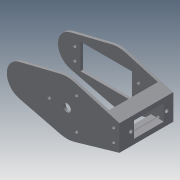
# Autodesk Inventor part: zakonceni_ramene
Saved by Autodesk Inventor 2013 (Build 170138000, 138)
## iProperties
Created: 2013-05-11
Part Number: zakonceni_ramene
Material: Generic
Document SubType Name: Modeling
Designer: idle-rug
Density: 1 g/cm^3
Author: idle-rug
Autodesk Inventor part; units mm, degrees
ref_plane "YZ Plane" through (0, 0, 0) normal (1, 0, 0) x (0, 1, 0)
ref_plane "XZ Plane" through (0, 0, 0) normal (0, 1, 0) x (-1, 0, 0)
ref_plane "XY Plane" through (0, 0, 0) normal (0, 0, 1) x (1, 0, 0)
sketch "Sketch1" plane through (0, 0, 0) normal (0, 1, 0) x (-1, 0, 0)
  circle A0 centre (0, 0) radius 21
  line L0 (-21, 0) -> (-41, 0)
  line L1 (-41, 0) -> (-41, -10)
  line L2 (-41, -10) -> (-18.466185, -10)
  line L3 (-41, 0) -> (-41, 10)
  line L4 (-41, 10) -> (-18.466185, 10)
  line L5 (-41, 10) -> (-5.8359, 20.17281)
  line L6 (-41, -10) -> (-5.8359, -20.17281)
  arc A1 (-5.8359, 20.17281) -> (-5.8359, -20.17281) centre (0, 0) ccw
  dimension "d0" = 42
  dimension "d1" = 20
  dimension "d2" = 10
  dimension "d3" = 10
  constraints: 14 end point, 7 point on circle, 4 tangent, 3 perpendicular, 2 centre point, 1 coincident, 1 horizontal, 1 parallel
  measures "d0" diameter of A0
  measures "d1" distance of L0.start L0.end
  measures "d2" distance of L0.end L1.end
  measures "d3" distance of L0.end L3.end
extrude "Extrusion1" add sketch "Sketch1" along normal blind 2
sketch "Sketch2" plane through (0, 0, 0) normal (0, -1, 0) x (1, 0, 0)
  arc A0 (5.8359, 20.17281) -> (5.8359, -20.17281) centre (0, 0) ccw
  circle A1 centre (0, 0) radius 3
  dimension "d11" = 6
  constraints: 1 centre point, 1 coincident
  measures "d11" diameter of A1
extrude "Extrusion2" cut sketch "Sketch2" against normal blind 2
sketch "Sketch3" plane through (0, 2, 0) normal (0, 1, 0) x (1, 0, 0)
  line L0 (5.8359, -20.17281) -> (41, -10)
  line L1 (41, -10) -> (41, 10)
  line L2 (41, 10) -> (5.8359, 20.17281)
  line L3 (39, 0) -> (39, 10.578591)
  line L4 (39, 0) -> (39, -10.578591)
  line L5 (41, 10) -> (41, -10)
  line L6 (39, -10.578591) -> (41, -10)
  line L7 (39, 10.578591) -> (41, 10)
  constraints: 10 end point, 3 collinear, 2 point on line, 1 parallel
extrude "Extrusion3" add sketch "Sketch3" along normal blind 48
sketch "Sketch4" plane through (0, 50, 0) normal (0, 1, 0) x (1, 0, 0)
  line L0 (41, -10) -> (41, 10)
  line L1 (39, -10.578591) -> (41, -10)
  circle A0 centre (0, 0) radius 21
  line L2 (41, 10) -> (5.8359, 20.17281)
  line L3 (41, -10) -> (5.8359, -20.17281)
  line L4 (41, 10) -> (41, -10)
  circle A1 centre (0, 0) radius 3
  dimension "d17" = 42
  dimension "d18" = 6
  constraints: 6 end point, 2 centre point, 2 coincident, 2 collinear, 2 point on circle, 1 tangent
  measures "d17" diameter of A0
  measures "d18" diameter of A1
extrude "Extrusion4" add sketch "Sketch4" along normal blind 2
sketch "Sketch5" plane through (41, 0, 10) normal (1, 0, 0) x (0, 0, -1)
  line L0 (10, 26) -> (10, 42)
  line L1 (10, 42) -> (10, 10)
  line L2 (10, 42) -> (10, 39.95)
  line L3 (10, 10) -> (10, 12.05)
  circle A0 centre (10, 39.95) radius 1.5
  circle A1 centre (10, 12.05) radius 1.5
  line L4 (10, 12.05) -> (10, 14.4)
  line L5 (10, 39.95) -> (10, 37.6)
  line L6 (10, 37.6) -> (10, 14.4)
  line L7 (16.2, 14.4) -> (3.8, 14.4)
  line L8 (3.8, 14.4) -> (3.8, 37.6)
  line L9 (3.8, 37.6) -> (16.2, 37.6)
  line L10 (16.2, 37.6) -> (16.2, 14.4)
  line L11 (16.2, 14.4) -> (3.8, 37.6) construction
  line L12 (3.8, 14.4) -> (16.2, 37.6) construction
  point P0 (10, 0)
  dimension "d23" = 2.05
  dimension "d24" = 2.05
  dimension "d25" = 3
  dimension "d26" = 3
  dimension "d27" = 2.35
  dimension "d28" = 2.35
  dimension "d29" = 12.4
  constraints: 26 end point, 4 point on line, 2 centre point, 2 coincident, 2 collinear, 2 midpoint, 2 parallel, 1 horizontal, 1 perpendicular
  measures "d23" distance of L0.end L2.end
  measures "d24" distance of L1.end L3.end
  measures "d25" diameter of A0
  measures "d26" diameter of A1
  measures "d27" distance of L4.start L4.end
  measures "d28" distance of L5.start L5.end
  measures "d29" distance of L8.end L9.end
extrude "Extrusion5" cut sketch "Sketch5" against normal blind 2
sketch "Sketch6" plane through (0, 52, 0) normal (0, 1, 0) x (1, 0, 0)
  arc A0 (5.8359, 20.17281) -> (5.8359, -20.17281) centre (0, 0) ccw
  circle A1 centre (-14.25, 0) radius 1.5
  line L0 (0, 0) -> (7.125, 12.340862)
  line L1 (0, 0) -> (14.25, 0) construction
  line L2 (0, 0) -> (7.125, -12.340862)
  line L3 (0, 0) -> (14.25, 0) construction
  circle A2 centre (7.125, 12.340862) radius 1.5
  circle A3 centre (7.125, -12.340862) radius 1.5
  dimension "d33" = 3
  dimension "d34" = 60
  dimension "d35" = 60
  dimension "d36" = 3
  dimension "d37" = 3
  constraints: 8 end point, 3 centre point, 3 coincident, 2 equal length, 2 horizontal
  measures "d33" diameter of A1
  measures "d34" angle of L1 L0
  measures "d35" angle of L2 L3
  measures "d36" diameter of A2
  measures "d37" diameter of A3
extrude "Extrusion6" cut sketch "Sketch6" against normal blind 2
sketch "Sketch7" plane through (0, 52, 0) normal (0, 1, 0) x (1, 0, 0)
  circle A0 centre (7.125, 12.340862) radius 1.5
  circle A1 centre (-14.25, 0) radius 1.5
  circle A2 centre (7.125, -12.340862) radius 1.5
  circle A3 centre (0, 0) radius 3
  line L0 (41, -10) -> (41, 10)
  line L1 (41, 10) -> (5.8359, 20.17281)
  arc A4 (5.8359, 20.17281) -> (5.8359, -20.17281) centre (0, 0) ccw
  line L2 (5.8359, -20.17281) -> (41, -10)
extrude "Extrusion7" cut sketch "Sketch7" against normal blind 1
sketch "Sketch8" plane through (0, 0, 0) normal (0, -1, 0) x (1, 0, 0)
  circle A0 centre (0, 0) radius 3
  line L0 (5.8359, 20.17281) -> (41, 10)
  arc A1 (5.8359, 20.17281) -> (5.8359, -20.17281) centre (0, 0) ccw
  line L1 (41, -10) -> (5.8359, -20.17281)
  line L2 (41, 10) -> (41, -10)
extrude "Extrusion8" cut sketch "Sketch8" against normal blind 1
sketch "Sketch9" plane through (0, 50, 0) normal (0, -1, 0) x (1, 0, 0)
  circle A0 centre (7.125, -12.340862) radius 1.5
  circle A1 centre (-14.25, 0) radius 1.5
  circle A2 centre (7.125, 12.340862) radius 1.5
  line L0 (39, -10.578591) -> (39, 10.578591)
  line L1 (5.8359, 20.17281) -> (39, 10.578591)
  arc A3 (5.8359, 20.17281) -> (5.8359, -20.17281) centre (0, 0) ccw
  line L2 (39, -10.578591) -> (5.8359, -20.17281)
  circle A4 centre (0, 0) radius 3
extrude "Extrusion9" add sketch "Sketch9" along normal blind 1
sketch "Sketch10" plane through (0, 2, 0) normal (0, 1, 0) x (1, 0, 0)
  line L0 (39, -10.578591) -> (39, 10.578591)
  line L1 (39, 10.578591) -> (5.8359, 20.17281)
  arc A0 (5.8359, 20.17281) -> (5.8359, -20.17281) centre (0, 0) ccw
  line L2 (5.8359, -20.17281) -> (39, -10.578591)
  circle A1 centre (0, 0) radius 3
extrude "Extrusion10" add sketch "Sketch10" along normal blind 1
sketch "Sketch11" plane through (0, 1, 0) normal (0, -1, 0) x (1, 0, 0)
  arc A0 (5.8359, 20.17281) -> (5.8359, -20.17281) centre (0, 0) ccw
  circle A1 centre (-14.25, 0) radius 1.5
  line L0 (0, 0) -> (14.25, 0) construction
  line L1 (0, 0) -> (14.25, 0) construction
  circle A2 centre (7.125, 12.340862) radius 1.5
  circle A3 centre (7.125, -12.340862) radius 1.5
  dimension "d52" = 3
  dimension "d53" = 3
  constraints: 4 end point, 3 centre point, 2 horizontal, 1 coincident
  measures "d52" diameter of A2
  measures "d53" diameter of A3
extrude "Extrusion11" cut sketch "Sketch11" against normal blind 2
sketch "Sketch12" plane through (0, 51, 0) normal (0, 1, 0) x (1, 0, 0)
  circle A0 centre (0, 0) radius 3
  circle A1 centre (-14.25, 0) radius 1.5
  line L0 (41, 10) -> (41, -10)
  arc A2 (5.8359, 20.17281) -> (5.8359, -20.17281) centre (0, 0) ccw
  line L1 (0, 0) -> (0, 21)
  line L2 (0, 0) -> (0, -21)
  line L3 (0, 0) -> (18.1, 0)
  line L4 (-36.9, 10) -> (18.1, 10)
  line L5 (18.1, 10) -> (18.1, -10)
  line L6 (18.1, -10) -> (-36.9, -10)
  line L7 (-36.9, -10) -> (-36.9, 10)
  line L8 (-46.9, 10) -> (-5.057146, 20.381984)
  line L9 (-46.9, 10) -> (-46.9, -10)
  line L10 (-46.9, -10) -> (-5.057146, -20.381984)
  arc A3 (-5.057146, 20.381984) -> (-5.057146, -20.381984) centre (0, 0) ccw
  line L11 (10.7, 10) -> (-29.5, 10)
  line L12 (-29.5, 10) -> (-29.5, -10)
  line L13 (-29.5, -10) -> (10.7, -10)
  line L14 (10.7, -10) -> (10.7, 10)
  line L15 (-29.5, 0) -> (-32.15, 0)
  line L16 (-29.5, 2.75) -> (-29.5, 0)
  line L17 (-29.5, 0) -> (-34.25, 0)
  line L18 (-29.5, 5.05) -> (-29.5, 0)
  circle A4 centre (-34.25, 5.05) radius 1.5
  circle A5 centre (-34.25, -5.05) radius 1.5
  circle A6 centre (15.45, 5.05) radius 1.5
  circle A7 centre (15.45, -5.05) radius 1.5
  point P0 (-9.4, 0)
  point P1 (-9.4, 0)
  dimension "d58" = 55
  dimension "d59" = 20
  dimension "d61" = 10
  dimension "d62" = 40.2
  dimension "d67" = 3
  dimension "d69" = 3
  dimension "d72" = 3
  dimension "d73" = 3
  constraints: 36 end point, 6 point on circle, 5 centre point, 5 parallel, 4 horizontal, 4 tangent, 3 perpendicular, 1 coincident, 1 collinear, 1 midpoint, 1 point on line
  measures "d58" distance of L5.end L6.end
  measures "d59" distance of L4.end L5.end
  measures "d61" distance of L4.start L8.start
  measures "d62" distance of L13.end L12.end
  measures "d67" diameter of A4
  measures "d69" diameter of A5
  measures "d72" diameter of A6
  measures "d73" diameter of A7
extrude "Extrusion12" add sketch "Sketch12" against normal blind 2 contours L3 L14 L6 L2 A0 | A0 L1 L4 L14 L3 | A0 L2 L6 A2 L4 L1 | L4 L7 L6 A2 L10 L9 L8 | A2 L6 L12 L4 | L12 L6 L7 L4 | A6 | A7
sketch "Sketch13" plane through (0, 51, 0) normal (0, 1, 0) x (1, 0, 0)
  circle A0 centre (15.45, 5.05) radius 1.5
  circle A1 centre (15.45, -5.05) radius 1.5
  dimension "d77" = 3
  dimension "d79" = 3
  constraints: 2 centre point
  measures "d77" diameter of A0
  measures "d79" diameter of A1
extrude "Extrusion13" cut sketch "Sketch13" against normal blind 2
sketch "Sketch14" plane through (0, 49, 0) normal (0, -1, 0) x (1, 0, 0)
  line L0 (-5.057146, 20.381984) -> (-46.9, 10)
  line L1 (-46.9, 10) -> (-46.9, -10)
  line L2 (-46.9, -10) -> (-5.057146, -20.381984)
  line L3 (-36.9, 0) -> (-36.9, 12.481184)
  line L4 (-36.9, 12.481184) -> (-46.9, 10)
  line L5 (-46.9, 10) -> (-46.9, -10)
  line L6 (-46.9, -10) -> (-36.9, -12.481184)
  line L7 (-36.9, -12.481184) -> (-36.9, 0)
  line L8 (-36.9, 12.481184) -> (-36.9, -12.481184)
  constraints: 12 end point, 3 collinear, 2 point on line, 1 parallel
extrude "Extrusion14" add sketch "Sketch14" along normal blind 46
sketch "Sketch15" plane through (0, 1, 0) normal (0, -1, 0) x (1, 0, 0)
  arc A0 (5.8359, 20.17281) -> (5.8359, -20.17281) centre (0, 0) ccw
  arc A1 (-5.071838, 20.378333) -> (-5.071838, -20.378333) centre (0, 0) ccw
  line L0 (-36.9, 0) -> (-34.25, 0)
  circle A2 centre (-34.25, 4.95) radius 1.5
  circle A3 centre (-34.25, -4.95) radius 1.5
  line L1 (18.1, 0) -> (15.45, 0)
  circle A4 centre (15.45, 4.95) radius 1.5
  circle A5 centre (15.45, -4.95) radius 1.5
  dimension "d85" = 18.1
  dimension "d87" = 2.65
  dimension "d108" = 3
  dimension "d109" = 3
  dimension "d110" = 2.65
  dimension "d112" = 3
  dimension "d113" = 3
  constraints: 5 centre point, 4 end point, 4 point on circle
  measures "d85" distance of A1.centre L1.start
  measures "d87" distance of L0.start L0.end
  measures "d108" diameter of A2
  measures "d109" diameter of A3
  measures "d110" distance of L1.start L1.end
  measures "d112" diameter of A4
  measures "d113" diameter of A5
sketch "Sketch16" plane through (0, 51, 0) normal (0, 1, 0) x (1, 0, 0)
  circle A0 centre (15.45, 5.05) radius 1.5
  circle A1 centre (15.45, -5.05) radius 1.5
  circle A2 centre (-34.25, -5.05) radius 1.5
  circle A3 centre (-34.25, 5.05) radius 1.5
  line L0 (-46.9, 10) -> (-46.9, -10)
  line L1 (15.45, 5.05) -> (15.45, 0)
  line L2 (15.45, -5.05) -> (15.45, 0)
  arc A4 (13.984921, -4.728218) -> (16.915079, -4.728218) centre (15.45, -5.05) ccw
  arc A5 (16.915079, 4.728218) -> (13.984921, 4.728218) centre (15.45, 5.05) ccw
  arc A6 (16.915079, 4.728218) -> (13.984921, 4.728218) centre (15.45, 0) ccw
  circle A7 centre (15.45, -4.95) radius 1.5
  circle A8 centre (15.45, 4.95) radius 1.5
  line L3 (-34.25, -5.05) -> (-34.25, 0)
  line L4 (-34.25, 5.05) -> (-34.25, 0)
  circle A9 centre (-34.25, -4.95) radius 1.5
  circle A10 centre (-34.25, 4.95) radius 1.5
  dimension "d92" = 3
  dimension "d93" = 3
  dimension "d95" = 3
  dimension "d96" = 3
  constraints: 11 point on circle, 8 end point, 7 centre point, 3 point on line, 2 collinear, 2 concentric, 2 parallel
  measures "d92" diameter of A7
  measures "d93" diameter of A8
  measures "d95" diameter of A9
  measures "d96" diameter of A10
extrude "Extrusion15" cut sketch "Sketch16" against normal blind 2 contours A8 A0 A6 | A0 L1 A8 | A8 L1 A0 | A6 L1 A0 | A0 L1 A6 | A7 A1 | A1 L2 A7 | A7 L2 A1 | A9 A2 | A2 L3 A9 | A9 L3 A2 | A10 A3 | A3 L4 A10 | A10 L4 A3 picked at (15.45, -5.476348) picked at (-34.25, -5.476348) picked at (-34.25, 5.476348)
sketch "Sketch17" plane through (0, 51, 0) normal (0, 1, 0) x (1, 0, 0)
  arc A0 (13.950834, 5) -> (16.949166, 5) centre (15.45, 4.95) ccw
  arc A1 (16.949166, -5) -> (13.950834, -5) centre (15.45, -4.95) ccw
  arc A2 (-32.750834, -5) -> (-35.749166, -5) centre (-34.25, -4.95) ccw
  arc A3 (-35.749166, 5) -> (-32.750834, 5) centre (-34.25, 4.95) ccw
  circle A4 centre (15.45, 4.95) radius 3.090834
  circle A5 centre (15.45, -4.95) radius 2.457153
  circle A6 centre (-34.25, 4.95) radius 2.908011
  circle A7 centre (-34.25, -4.95) radius 2.355897
  constraints: 4 centre point, 4 coincident
extrude "Extrusion16" cut sketch "Sketch17" against normal blind 2
sketch "Sketch18" plane through (0, 51, 0) normal (0, 1, 0) x (1, 0, 0)
  circle A0 centre (-34.25, 4.95) radius 2.908011
  circle A1 centre (-34.25, -4.95) radius 2.355897
  circle A2 centre (15.45, -4.95) radius 2.457153
  circle A3 centre (15.45, 4.95) radius 3.090834
  circle A4 centre (-34.25, 4.95) radius 1.5
  circle A5 centre (-34.25, -4.95) radius 1.5
  circle A6 centre (15.45, 4.95) radius 1.5
  circle A7 centre (15.45, -4.95) radius 1.5
  dimension "d101" = 3
  dimension "d102" = 3
  dimension "d103" = 3
  dimension "d104" = 3
  constraints: 4 centre point, 4 coincident
  measures "d101" diameter of A4
  measures "d102" diameter of A5
  measures "d103" diameter of A6
  measures "d104" diameter of A7
extrude "Extrusion17" add sketch "Sketch18" against normal blind 2
sketch "Sketch19" plane through (0, 1, 0) normal (0, -1, 0) x (1, 0, 0)
  arc A0 (5.8359, 20.17281) -> (5.8359, -20.17281) centre (0, 0) ccw
  line L0 (41, 10) -> (41, -10)
  line L1 (0, 0) -> (18.1, 0)
  line L2 (18.1, 0) -> (-46.9, 0)
  line L3 (-46.9, 0) -> (-46.9, 10)
  line L4 (-46.9, 0) -> (-46.9, -10)
  line L5 (-46.9, 10) -> (-5.057146, 20.381984)
  line L6 (-46.9, -10) -> (-5.057146, -20.381984)
  arc A1 (-5.057146, 20.381984) -> (-5.057146, -20.381984) centre (0, 0) ccw
  dimension "d114" = 18.1
  dimension "d115" = 65
  constraints: 12 end point, 4 point on circle, 4 tangent, 2 perpendicular, 1 centre point, 1 collinear, 1 point on line
  measures "d114" distance of L1.start L1.end
  measures "d115" distance of L1.end L2.end
extrude "Extrusion18" add sketch "Sketch19" against normal blind 2
extrude "Extrusion19" cut sketch "Sketch15" against normal blind 2
sketch "Sketch21" plane through (39, 49, -10.578591) normal (-1, 0, 0) x (0, 0, 1)
  line L0 (0, -46) -> (21.157181, -46)
  line L1 (21.157181, -46) -> (21.157181, 0)
  line L2 (21.157181, 0) -> (0, 0)
  line L3 (0, -46) -> (0, 0)
  line L4 (4.378591, -34.6) -> (4.378591, -11.4)
  line L5 (4.378591, -11.4) -> (16.778591, -11.4)
  line L6 (16.778591, -11.4) -> (16.778591, -34.6)
  line L7 (16.778591, -34.6) -> (4.378591, -34.6)
  circle A0 centre (10.578591, -9.05) radius 1.5
  circle A1 centre (10.578591, -36.95) radius 1.5
  point P0 (10.578591, -49)
extrude "Extrusion20" add sketch "Sketch21" along normal blind 8
sketch "Sketch22" plane through (0, 49, 0) normal (0, -1, 0) x (1, 0, 0)
  line L0 (39, -10.578591) -> (31, -10.578591)
  line L1 (31, 10.578591) -> (39, 10.578591)
  line L2 (39, 10.578591) -> (5.8359, 20.17281)
  line L3 (-36.9, 12.481184) -> (-36.9, -12.481184)
  line L4 (5.8359, -20.17281) -> (39, -10.578591)
  line L5 (31, -10.578591) -> (31, -12.892953)
  line L6 (31, -12.892953) -> (39, -10.578591)
  line L7 (39, -10.578591) -> (31, -10.578591)
  line L8 (31, 10.578591) -> (31, 12.892953)
  line L9 (31, 12.892953) -> (39, 10.578591)
  line L10 (39, 10.578591) -> (31, 10.578591)
  constraints: 12 end point, 4 collinear, 2 point on line, 1 parallel, 1 perpendicular
extrude "Extrusion21" add sketch "Sketch22" along normal blind 46
sketch "Sketch23" plane through (0, 51, 0) normal (0, 1, 0) x (1, 0, 0)
  line L0 (10.7, 10) -> (-29.5, 10)
  line L1 (-29.5, 10) -> (-29.5, -10)
  line L2 (-29.5, -10) -> (10.7, -10)
  line L3 (10.7, -10) -> (10.7, 10)
  dimension "d131" = 40.2
  constraints: 8 end point, 2 parallel, 1 horizontal, 1 perpendicular
  measures "d131" distance of L2.end L1.end
extrude "Extrusion22" cut sketch "Sketch23" against normal blind 2
sketch "Sketch24" plane through (0, 1, 0) normal (0, -1, 0) x (1, 0, 0)
  circle A0 centre (15.45, 4.95) radius 1.5 projected
  circle A1 centre (-34.25, 4.95) radius 1.5 projected
  circle A2 centre (-34.25, -4.95) radius 1.5 projected
  circle A3 centre (15.45, -4.95) radius 1.5 projected
extrude "Extrusion23" add sketch "Sketch24" against normal blind 2
sketch "Sketch25" plane through (0, 51, 0) normal (0, 1, 0) x (1, 0, 0)
  circle A0 centre (7.125, 12.340862) radius 1.5
  circle A1 centre (7.125, -12.340862) radius 1.5
extrude "Extrusion24" add sketch "Sketch25" against normal blind 2
sketch "Sketch26" plane through (0, 3, 0) normal (0, 1, 0) x (1, 0, 0)
  line L0 (31, -12.892953) -> (31, 12.892953)
  line L1 (31, 12.892953) -> (5.8359, 20.17281)
  arc A0 (5.8359, 20.17281) -> (-5.057146, 20.381984) centre (0, 0) ccw
  line L2 (-5.057146, 20.381984) -> (-36.9, 12.481184)
  line L3 (-36.9, 12.481184) -> (-36.9, -12.481184)
  line L4 (-36.9, -12.481184) -> (-5.057146, -20.381984)
  arc A1 (-5.057146, -20.381984) -> (5.8359, -20.17281) centre (0, 0) ccw
  line L5 (5.8359, -20.17281) -> (31, -12.892953)
  circle A2 centre (7.125, -12.340862) radius 1.5
  circle A3 centre (-14.25, 0) radius 1.5
  circle A4 centre (7.125, 12.340862) radius 1.5
  circle A5 centre (0, 0) radius 3
extrude "Extrusion25" add sketch "Sketch26" along normal blind 4
sketch "Sketch27" plane through (0, 49, 0) normal (0, -1, 0) x (1, 0, 0)
  line L0 (-29.5, -10) -> (-29.5, 10)
  line L1 (-29.5, 10) -> (10.7, 10)
  line L2 (10.7, 10) -> (10.7, -10)
  line L3 (10.7, -10) -> (-29.5, -10)
  circle A0 centre (-34.25, -4.95) radius 1.5
  circle A1 centre (-34.25, 4.95) radius 1.5
  circle A2 centre (15.45, 4.95) radius 1.5
  circle A3 centre (15.45, -4.95) radius 1.5
  line L4 (31, -12.892953) -> (31, 12.892953)
  line L5 (31, 12.892953) -> (5.8359, 20.17281)
  arc A4 (5.8359, 20.17281) -> (-5.057146, 20.381984) centre (0, 0) ccw
  line L6 (-5.057146, 20.381984) -> (-36.9, 12.481184)
  line L7 (-36.9, 12.481184) -> (-36.9, -12.481184)
  line L8 (-36.9, -12.481184) -> (-5.057146, -20.381984)
  arc A5 (-5.057146, -20.381984) -> (5.8359, -20.17281) centre (0, 0) ccw
  line L9 (5.8359, -20.17281) -> (31, -12.892953)
extrude "Extrusion26" add sketch "Sketch27" along normal blind 4
sketch "Sketch28" plane through (0, 1, 0) normal (0, -1, 0) x (1, 0, 0)
  circle A0 centre (7.125, 12.340862) radius 1.5
  circle A1 centre (-14.25, 0) radius 1.5
  circle A2 centre (7.125, -12.340862) radius 1.5
  circle A3 centre (0, 0) radius 3
  line L0 (5.8359, 20.17281) -> (41, 10)
  arc A4 (5.8359, 20.17281) -> (-5.057146, 20.381984) centre (0, 0) ccw
  line L1 (-5.057146, 20.381984) -> (-46.9, 10)
  line L2 (-46.9, 10) -> (-46.9, -10)
  line L3 (-46.9, -10) -> (-5.057146, -20.381984)
  arc A5 (-5.057146, -20.381984) -> (5.8359, -20.17281) centre (0, 0) ccw
  line L4 (41, -10) -> (5.8359, -20.17281)
  line L5 (41, 10) -> (41, -10)
extrude "Extrusion27" cut sketch "Sketch28" against normal blind 4
sketch "Sketch29" plane through (0, 51, 0) normal (0, 1, 0) x (1, 0, 0)
  line L0 (-29.5, -10) -> (-29.5, 10)
  line L1 (-29.5, 10) -> (10.7, 10)
  line L2 (10.7, 10) -> (10.7, -10)
  line L3 (10.7, -10) -> (-29.5, -10)
  circle A0 centre (-34.25, 4.95) radius 1.5
  circle A1 centre (-34.25, -4.95) radius 1.5
  circle A2 centre (15.45, -4.95) radius 1.5
  circle A3 centre (15.45, 4.95) radius 1.5
  arc A4 (-5.057146, -20.381984) -> (5.8359, -20.17281) centre (0, 0) ccw
  line L4 (41, -10) -> (5.8359, -20.17281)
  line L5 (41, 10) -> (41, -10)
  line L6 (5.8359, 20.17281) -> (41, 10)
  arc A5 (5.8359, 20.17281) -> (-5.057146, 20.381984) centre (0, 0) ccw
  line L7 (-5.057146, 20.381984) -> (-46.9, 10)
  line L8 (-46.9, 10) -> (-46.9, -10)
  line L9 (-46.9, -10) -> (-5.057146, -20.381984)
extrude "Extrusion28" cut sketch "Sketch29" against normal blind 4
sketch "Sketch30" plane through (-36.9, 7, 12.481184) normal (1, 0, 0) x (0, 0, -1)
  line L0 (24.962369, 38) -> (0, 38)
  line L1 (0, 38) -> (0, 0)
  line L2 (0, 0) -> (24.962369, 0)
  line L3 (24.962369, 38) -> (24.962369, 0)
  point P0 (12.481184, -7)
extrude "Extrusion29" cut sketch "Sketch30" against normal blind 10
sketch "Sketch31" plane through (41, 5, 10) normal (1, 0, 0) x (0, 0, -1)
  line L0 (16.2, 32.6) -> (16.2, 9.4) projected
  line L1 (16.2, 9.4) -> (3.8, 9.4) projected
  line L2 (3.8, 9.4) -> (3.8, 32.6) projected
  line L3 (3.8, 32.6) -> (16.2, 32.6) projected
  circle A0 centre (10, 34.95) radius 1.5 projected
  circle A1 centre (10, 7.05) radius 1.5 projected
  point P0 (10, -5)
extrude "Extrusion30" add sketch "Sketch31" against normal blind 10
sketch "Sketch32" plane through (41, 5, 10) normal (1, 0, 0) x (0, 0, -1)
  line L0 (0, 0) -> (0, 42) projected
  line L1 (20, 0) -> (20, 42) projected
  line L2 (0, 42) -> (0, 40)
  line L3 (0, 40) -> (20, 40)
  line L4 (0, 0) -> (0, 2)
  line L5 (0, 2) -> (20, 2)
  line L6 (10, 2) -> (10, 40)
  line L7 (10, 5) -> (10, 9.1)
  circle A0 centre (10, 37) radius 1.5
  circle A1 centre (10, 9.1) radius 1.5
  line L8 (10, 9.1) -> (10, 37)
  line L9 (3.8, 34.65) -> (16.2, 34.65)
  line L10 (16.2, 34.65) -> (16.2, 11.45)
  line L11 (16.2, 11.45) -> (3.8, 11.45)
  line L12 (3.8, 11.45) -> (3.8, 34.65)
  line L13 (3.8, 34.65) -> (16.2, 11.45) construction
  line L14 (16.2, 34.65) -> (3.8, 11.45) construction
  point P0 (10, -5)
  point P1 (10, 23.05)
  dimension "d150" = 2
  dimension "d153" = 2
  dimension "d161" = 4.1
  dimension "d163" = 3
  dimension "d164" = 3
  dimension "d165" = 12.4
  dimension "d166" = 23.2
  constraints: 26 end point, 7 point on line, 5 midpoint, 3 perpendicular, 2 centre point, 2 parallel, 1 coincident, 1 collinear, 1 horizontal
  measures "d150" distance of L0.end L2.end
  measures "d153" distance of L0.start L4.end
  measures "d161" distance of L7.start L7.end
  measures "d163" diameter of A0
  measures "d164" diameter of A1
  measures "d165" distance of L10.end L11.end
  measures "d166" distance of L9.end L10.end
extrude "Extrusion31" cut sketch "Sketch32" against normal blind 10 contours A0 L6 | L6 A0 | A1 L6 | L6 A1 | L9 L10 L11 L6 | L6 L11 L12 L9
sketch "Sketch33" plane through (0, 5, 0) normal (0, -1, 0) x (1, 0, 0)
  circle A0 centre (36, 5) radius 1.5
  circle A1 centre (36, -5) radius 1.5
  dimension "d170" = 3
  dimension "d171" = 3
  constraints: 2 centre point
  measures "d170" diameter of A0
  measures "d171" diameter of A1
extrude "Extrusion32" cut sketch "Sketch33" against normal blind 42
sketch "Sketch34" plane through (0, 47, 0) normal (0, 1, 0) x (1, 0, 0)
  circle A0 centre (-34.25, -4.95) radius 1.5
  circle A1 centre (-34.25, 4.95) radius 1.5
  line L0 (-5.057146, -20.381984) -> (-46.9, -10)
  circle A2 centre (-34.25, 0) radius 12.752035
  constraints: 1 centre point, 1 tangent
extrude "Extrusion33" cut sketch "Sketch34" against normal blind 2
sketch "Sketch35" plane through (0, 47, 0) normal (0, 1, 0) x (1, 0, 0)
  arc A0 (-46.9, -1.609939) -> (-37.3209, -12.376751) centre (-34.25, 0) ccw
  line L0 (-46.9, -10) -> (-46.9, -1.609939)
  line L1 (-37.3209, -12.376751) -> (-46.9, -10)
  point P0 (0, 0)
extrude "Extrusion34" cut sketch "Sketch35" against normal blind 2
sketch "Sketch36" plane through (0, 47, 0) normal (0, 1, 0) x (1, 0, 0)
  arc A0 (-37.3209, 12.376751) -> (-46.9, 1.609939) centre (-34.25, 0) ccw
  line L0 (-46.9, 10) -> (-37.3209, 12.376751)
  line L1 (-46.9, 1.609939) -> (-46.9, 10)
  point P0 (0, 0)
extrude "Extrusion35" cut sketch "Sketch36" against normal blind 2
sketch "Sketch37" plane through (0, 47, 0) normal (0, 1, 0) x (1, 0, 0)
  arc A0 (-26.337074, 10) -> (-37.3209, 12.376751) centre (-34.25, 0) ccw
  line L0 (10.7, 10) -> (-26.337074, 10)
  line L1 (10.7, -10) -> (10.7, 10)
  line L2 (-26.337074, -10) -> (10.7, -10)
  arc A1 (-37.3209, -12.376751) -> (-26.337074, -10) centre (-34.25, 0) ccw
  arc A2 (-37.3209, 12.376751) -> (-37.3209, -12.376751) centre (-34.25, 0) ccw
  line L3 (10.7, -10) -> (-29.5, -10)
  line L4 (-29.5, -10) -> (-29.5, 10)
  line L5 (-29.5, 10) -> (10.7, 10)
  line L6 (10.7, 10) -> (10.7, -10)
  circle A3 centre (-34.25, 4.95) radius 1.5
  circle A4 centre (-34.25, -4.95) radius 1.5
  dimension "d180" = 40.2
  dimension "d183" = 3
  dimension "d184" = 3
  constraints: 8 end point, 3 centre point, 2 concentric, 2 parallel, 2 point on circle, 1 horizontal, 1 perpendicular, 1 point on line
  measures "d180" distance of L4.end L5.end
  measures "d183" diameter of A3
  measures "d184" diameter of A4
extrude "Extrusion36" add sketch "Sketch37" against normal blind 2 contours L5 L4 L3 A1 A2 A0
sketch "Sketch38" plane through (0, 5, 0) normal (0, -1, 0) x (1, 0, 0)
  line L0 (-46.9, 10) -> (-5.057146, 20.381984)
  line L1 (-46.9, -10) -> (-46.9, 10)
  arc A0 (-5.057146, -20.381984) -> (5.8359, -20.17281) centre (0, 0) ccw
  line L2 (0, 0) -> (-34.25, 0)
  circle A1 centre (-34.25, 0) radius 12.752035
  dimension "d187" = 34.25
  constraints: 2 end point, 1 centre point, 1 coincident, 1 perpendicular, 1 tangent
  measures "d187" distance of L2.start L2.end
extrude "Extrusion37" cut sketch "Sketch38" against normal blind 2 contours A1 L1 | L1 A1
sketch "Sketch39" plane through (0, 5, 0) normal (0, -1, 0) x (1, 0, 0)
  arc A0 (-46.9, -1.609939) -> (-37.3209, -12.376751) centre (-34.25, 0) ccw
  line L0 (-46.9, -10) -> (-46.9, -1.609939)
  line L1 (-37.3209, -12.376751) -> (-46.9, -10)
  point P0 (0, 0)
extrude "Extrusion38" cut sketch "Sketch39" against normal blind 2
sketch "Sketch40" plane through (0, 5, 0) normal (0, -1, 0) x (1, 0, 0)
  arc A0 (-37.3209, 12.376751) -> (-46.9, 1.609939) centre (-34.25, 0) ccw
  line L0 (-46.9, 10) -> (-37.3209, 12.376751)
  line L1 (-46.9, 1.609939) -> (-46.9, 10)
  point P0 (0, 0)
extrude "Extrusion39" cut sketch "Sketch40" against normal blind 2
sketch "Sketch41" plane through (0, 5, 0) normal (0, -1, 0) x (1, 0, 0)
  arc A0 (-37.3209, -12.376751) -> (-37.3209, 12.376751) centre (-34.25, 0) ccw
  circle A1 centre (-34.25, 0) radius 12.752035
  constraints: 1 coincident, 3 other
extrude "Extrusion40" add sketch "Sketch41" against normal blind 2
body "Solid1"
